Autodesk Inventor part; units mm, degrees
(part 2 of 2)
sketch "Sketch7" plane through (0, 0, 5.08) normal (0, 0, 1) x (1, 0, 0)
  circle A0 centre (7.62, 538.4546) radius 2.5 projected
  circle A1 centre (7.62, 482.5746) radius 2.5 projected
  line L0 (213.36, 469.8746) -> (213.36, 464.7946) projected
  line L1 (213.36, 464.7946) -> (203.2, 464.7946) projected
  line L2 (203.2, 464.7946) -> (203.2, 469.8746) projected
  line L3 (203.2, 469.8746) -> (213.36, 469.8746) projected
  line L4 (172.72, 469.8746) -> (172.72, 464.7946) projected
  line L5 (172.72, 464.7946) -> (162.56, 464.7946) projected
  line L6 (162.56, 464.7946) -> (162.56, 469.8746) projected
  line L7 (162.56, 469.8746) -> (172.72, 469.8746) projected
  line L8 (193.04, 469.8746) -> (193.04, 464.7946) projected
  line L9 (193.04, 464.7946) -> (182.88, 464.7946) projected
  line L10 (182.88, 464.7946) -> (182.88, 469.8746) projected
  line L11 (182.88, 469.8746) -> (193.04, 469.8746) projected
  line L12 (233.68, 469.8746) -> (233.68, 464.7946) projected
  line L13 (233.68, 464.7946) -> (223.52, 464.7946) projected
  line L14 (223.52, 464.7946) -> (223.52, 469.8746) projected
  line L15 (223.52, 469.8746) -> (233.68, 469.8746) projected
  line L16 (228.6, 71.1074) -> (223.52, 71.1074) projected
  line L17 (228.6, 60.9474) -> (228.6, 71.1074) projected
  line L18 (223.52, 60.9474) -> (228.6, 60.9474) projected
  line L19 (223.52, 60.9474) -> (223.52, 50.7874) projected
  line L20 (228.6, 50.7874) -> (223.52, 50.7874) projected
  line L21 (228.6, 40.6274) -> (228.6, 50.7874) projected
  line L22 (223.52, 40.6274) -> (228.6, 40.6274) projected
  line L23 (223.52, 40.6274) -> (223.52, 30.4674) projected
  line L24 (228.6, 30.4674) -> (223.52, 30.4674) projected
  line L25 (228.6, 20.3074) -> (228.6, 30.4674) projected
  line L26 (223.52, 20.3074) -> (228.6, 20.3074) projected
  line L27 (223.52, 20.3074) -> (223.52, 10.1474) projected
  line L28 (228.6, 10.1474) -> (223.52, 10.1474) projected
  line L29 (228.6, 0) -> (228.6, 10.1474) projected
  line L30 (228.6, 0) -> (309.88, 0) projected
  line L31 (309.88, 10.1474) -> (309.88, 0) projected
  line L32 (314.96, 10.1474) -> (309.88, 10.1474) projected
  line L33 (314.96, 10.1474) -> (314.96, 20.3074) projected
  line L34 (309.88, 20.3074) -> (314.96, 20.3074) projected
  line L35 (309.88, 30.4674) -> (309.88, 20.3074) projected
  line L36 (314.96, 30.4674) -> (309.88, 30.4674) projected
  line L37 (314.96, 30.4674) -> (314.96, 40.6274) projected
  line L38 (309.88, 40.6274) -> (314.96, 40.6274) projected
  line L39 (309.88, 50.7874) -> (309.88, 40.6274) projected
  line L40 (314.96, 50.7874) -> (309.88, 50.7874) projected
  line L41 (314.96, 50.7874) -> (314.96, 60.9474) projected
  line L42 (309.88, 60.9474) -> (314.96, 60.9474) projected
  line L43 (309.88, 71.1074) -> (309.88, 60.9474) projected
  line L44 (314.96, 71.1074) -> (309.88, 71.1074) projected
  line L45 (314.96, 71.1074) -> (314.96, 81.2674) projected
  line L46 (314.96, 81.2674) -> (309.88, 81.2674) projected
  line L47 (309.88, 81.2674) -> (309.88, 91.4274) projected
  line L48 (309.88, 91.4274) -> (314.96, 91.4274) projected
  line L49 (314.96, 91.4274) -> (314.96, 101.5874) projected
  line L50 (314.96, 101.5874) -> (309.88, 101.5874) projected
  line L51 (309.88, 101.5874) -> (309.88, 111.7474) projected
  line L52 (309.88, 111.7474) -> (314.96, 111.7474) projected
  line L53 (314.96, 111.7474) -> (314.96, 121.9074) projected
  line L54 (314.96, 121.9074) -> (309.88, 121.9074) projected
  line L55 (309.88, 121.9074) -> (309.88, 132.0674) projected
  line L56 (309.88, 132.0674) -> (314.96, 132.0674) projected
  line L57 (314.96, 132.0674) -> (314.96, 142.2274) projected
  line L58 (314.96, 142.2274) -> (309.88, 142.2274) projected
  line L59 (309.88, 142.2274) -> (309.88, 152.3874) projected
  line L60 (309.88, 152.3874) -> (314.96, 152.3874) projected
  line L61 (314.96, 152.3874) -> (314.96, 162.5474) projected
  line L62 (314.96, 162.5474) -> (309.88, 162.5474) projected
  line L63 (309.88, 162.5474) -> (309.88, 172.7074) projected
  line L64 (309.88, 172.7074) -> (314.96, 172.7074) projected
  line L65 (314.96, 172.7074) -> (314.96, 182.8674) projected
  line L66 (314.96, 182.8674) -> (309.88, 182.8674) projected
  line L67 (309.88, 182.8674) -> (309.88, 193.0274) projected
  line L68 (309.88, 193.0274) -> (314.96, 193.0274) projected
  line L69 (314.96, 193.0274) -> (314.96, 203.1874) projected
  line L70 (314.96, 203.1874) -> (309.88, 203.1874) projected
  line L71 (309.88, 203.1874) -> (309.88, 213.3474) projected
  line L72 (309.88, 213.3474) -> (314.96, 213.3474) projected
  line L73 (314.96, 213.3474) -> (314.96, 223.5074) projected
  line L74 (314.96, 223.5074) -> (309.88, 223.5074) projected
  line L75 (309.88, 223.5074) -> (309.88, 233.6674) projected
  line L76 (309.88, 233.6674) -> (314.96, 233.6674) projected
  line L77 (314.96, 233.6674) -> (314.96, 243.8274) projected
  line L78 (314.96, 243.8274) -> (309.88, 243.8274) projected
  line L79 (309.88, 243.8274) -> (309.88, 253.9874) projected
  line L80 (309.88, 253.9874) -> (314.96, 253.9874) projected
  line L81 (314.96, 253.9874) -> (314.96, 264.1474) projected
  line L82 (314.96, 264.1474) -> (309.88, 264.1474) projected
  line L83 (309.88, 264.1474) -> (309.88, 274.3074) projected
  line L84 (309.88, 274.3074) -> (314.96, 274.3074) projected
  line L85 (314.96, 274.3074) -> (314.96, 284.4674) projected
  line L86 (314.96, 284.4674) -> (309.88, 284.4674) projected
  line L87 (309.88, 284.4674) -> (309.88, 294.6274) projected
  line L88 (309.88, 294.6274) -> (314.96, 294.6274) projected
  line L89 (314.96, 294.6274) -> (314.96, 304.7874) projected
  line L90 (314.96, 304.7874) -> (309.88, 304.7874) projected
  line L91 (309.88, 304.7874) -> (309.88, 314.9474) projected
  line L92 (309.88, 314.9474) -> (314.96, 314.9474) projected
  line L93 (314.96, 314.9474) -> (314.96, 325.1074) projected
  line L94 (314.96, 325.1074) -> (309.88, 325.1074) projected
  line L95 (309.88, 325.1074) -> (309.88, 335.2674) projected
  line L96 (309.88, 335.2674) -> (314.96, 335.2674) projected
  line L97 (314.96, 335.2674) -> (314.96, 345.4274) projected
  line L98 (314.96, 345.4274) -> (309.88, 345.4274) projected
  line L99 (309.88, 345.4274) -> (309.88, 355.5874) projected
  line L100 (309.88, 355.5874) -> (314.96, 355.5874) projected
  line L101 (314.96, 355.5874) -> (314.96, 365.7474) projected
  line L102 (314.96, 365.7474) -> (309.88, 365.7474) projected
  line L103 (309.88, 365.7474) -> (309.88, 375.9074) projected
  line L104 (309.88, 375.9074) -> (314.96, 375.9074) projected
  line L105 (314.96, 375.9074) -> (314.96, 386.0674) projected
  line L106 (314.96, 386.0674) -> (309.88, 386.0674) projected
  line L107 (309.88, 386.0674) -> (309.88, 396.2274) projected
  line L108 (309.88, 396.2274) -> (314.96, 396.2274) projected
  line L109 (314.96, 396.2274) -> (314.96, 434.1031) projected
  line L110 (314.96, 434.1031) -> (304.1837, 444.8794) projected
  line L111 (304.1837, 444.8794) -> (300.5916, 441.2873) projected
  line L112 (300.5916, 441.2873) -> (293.4074, 448.4715) projected
  line L113 (293.4074, 448.4715) -> (296.9995, 452.0636) projected
  line L114 (296.9995, 452.0636) -> (289.8153, 459.2478) projected
  line L115 (289.8153, 459.2478) -> (286.2232, 455.6557) projected
  line L116 (286.2232, 455.6557) -> (279.039, 462.8399) projected
  line L117 (279.039, 462.8399) -> (282.6311, 466.432) projected
  line L118 (282.6311, 466.432) -> (275.4469, 473.6162) projected
  line L119 (275.4469, 473.6162) -> (271.8548, 470.0241) projected
  line L120 (271.8548, 470.0241) -> (264.6706, 477.2083) projected
  line L121 (264.6706, 477.2083) -> (268.2627, 480.8004) projected
  line L122 (268.2627, 480.8004) -> (261.0785, 487.9847) projected
  line L123 (261.0785, 487.9847) -> (257.4864, 484.3926) projected
  line L124 (257.4864, 484.3926) -> (250.3022, 491.5768) projected
  line L125 (250.3022, 491.5768) -> (253.8943, 495.1689) projected
  line L126 (253.8943, 495.1689) -> (246.7101, 502.3531) projected
  line L127 (246.7101, 502.3531) -> (243.118, 498.761) projected
  line L128 (243.118, 498.761) -> (235.9337, 505.9452) projected
  line L129 (235.9337, 505.9452) -> (239.5258, 509.5373) projected
  line L130 (239.5258, 509.5373) -> (232.3416, 516.7215) projected
  line L131 (232.3416, 516.7215) -> (228.7495, 513.1294) projected
  line L132 (228.7495, 513.1294) -> (221.5653, 520.3136) projected
  line L133 (221.5653, 520.3136) -> (225.1574, 523.9057) projected
  line L134 (225.1574, 523.9057) -> (217.9732, 531.0899) projected
  line L135 (217.9732, 531.0899) -> (214.3811, 527.4978) projected
  line L136 (214.3811, 527.4978) -> (207.1969, 534.682) projected
  line L137 (207.1969, 534.682) -> (210.789, 538.2741) projected
  line L138 (210.789, 538.2741) -> (203.6048, 545.4583) projected
  line L139 (203.6048, 545.4583) -> (200.0127, 541.8662) projected
  line L140 (200.0127, 541.8662) -> (192.8285, 549.0504) projected
  line L141 (192.8285, 549.0504) -> (196.4206, 552.6425) projected
  line L142 (196.4206, 552.6425) -> (193.04, 556.0231) projected
  line L143 (193.04, 556.0231) -> (193.04, 551.1546) projected
  line L144 (193.04, 551.1546) -> (182.88, 551.1546) projected
  line L145 (182.88, 551.1546) -> (182.88, 556.2346) projected
  line L146 (182.88, 556.2346) -> (172.72, 556.2346) projected
  line L147 (172.72, 556.2346) -> (172.72, 551.1546) projected
  line L148 (172.72, 551.1546) -> (162.56, 551.1546) projected
  line L149 (162.56, 551.1546) -> (162.56, 556.2346) projected
  line L150 (162.56, 556.2346) -> (152.4, 556.2346) projected
  line L151 (152.4, 556.2346) -> (152.4, 551.1546) projected
  line L152 (152.4, 551.1546) -> (142.24, 551.1546) projected
  line L153 (142.24, 551.1546) -> (142.24, 556.2346) projected
  line L154 (142.24, 556.2346) -> (132.08, 556.2346) projected
  line L155 (132.08, 556.2346) -> (132.08, 551.1546) projected
  line L156 (132.08, 551.1546) -> (121.92, 551.1546) projected
  line L157 (121.92, 551.1546) -> (121.92, 556.2346) projected
  line L158 (121.92, 556.2346) -> (111.76, 556.2346) projected
  line L159 (111.76, 556.2346) -> (111.76, 551.1546) projected
  line L160 (111.76, 551.1546) -> (101.6, 551.1546) projected
  line L161 (101.6, 551.1546) -> (101.6, 556.2346) projected
  line L162 (101.6, 556.2346) -> (91.44, 556.2346) projected
  line L163 (91.44, 556.2346) -> (91.44, 551.1546) projected
  line L164 (91.44, 551.1546) -> (81.28, 551.1546) projected
  line L165 (81.28, 551.1546) -> (81.28, 556.2346) projected
  line L166 (81.28, 556.2346) -> (71.12, 556.2346) projected
  line L167 (71.12, 556.2346) -> (71.12, 551.1546) projected
  line L168 (71.12, 551.1546) -> (60.96, 551.1546) projected
  line L169 (60.96, 551.1546) -> (60.96, 556.2346) projected
  line L170 (60.96, 556.2346) -> (50.8, 556.2346) projected
  line L171 (50.8, 556.2346) -> (50.8, 551.1546) projected
  line L172 (50.8, 551.1546) -> (40.64, 551.1546) projected
  line L173 (40.64, 551.1546) -> (40.64, 556.2346) projected
  line L174 (40.64, 556.2346) -> (30.48, 556.2346) projected
  line L175 (30.48, 556.2346) -> (30.48, 551.1546) projected
  line L176 (30.48, 551.1546) -> (20.32, 551.1546) projected
  line L177 (20.32, 551.1546) -> (20.32, 556.2346) projected
  line L178 (20.32, 556.2346) -> (10.16, 556.2346) projected
  line L179 (10.16, 556.2346) -> (10.16, 551.1546) projected
  line L180 (10.16, 551.1546) -> (-5.08, 551.1546) projected
  line L181 (-5.08, 551.1546) -> (-5.08, 469.8746) projected
  line L182 (-5.08, 469.8746) -> (10.16, 469.8746) projected
  line L183 (10.16, 469.8746) -> (10.16, 464.7946) projected
  line L184 (10.16, 464.7946) -> (20.32, 464.7946) projected
  line L185 (20.32, 464.7946) -> (20.32, 469.8746) projected
  line L186 (20.32, 469.8746) -> (30.48, 469.8746) projected
  line L187 (30.48, 469.8746) -> (30.48, 464.7946) projected
  line L188 (30.48, 464.7946) -> (40.64, 464.7946) projected
  line L189 (40.64, 464.7946) -> (40.64, 469.8746) projected
  line L190 (40.64, 469.8746) -> (50.8, 469.8746) projected
  line L191 (50.8, 469.8746) -> (50.8, 464.7946) projected
  line L192 (50.8, 464.7946) -> (60.96, 464.7946) projected
  line L193 (60.96, 464.7946) -> (60.96, 469.8746) projected
  line L194 (60.96, 469.8746) -> (71.12, 469.8746) projected
  line L195 (71.12, 469.8746) -> (71.12, 464.7946) projected
  line L196 (71.12, 464.7946) -> (81.28, 464.7946) projected
  line L197 (81.28, 464.7946) -> (81.28, 469.8746) projected
  line L198 (81.28, 469.8746) -> (91.44, 469.8746) projected
  line L199 (91.44, 469.8746) -> (91.44, 464.7946) projected
  line L200 (91.44, 464.7946) -> (101.6, 464.7946) projected
  line L201 (101.6, 464.7946) -> (101.6, 469.8746) projected
  line L202 (101.6, 469.8746) -> (111.76, 469.8746) projected
  line L203 (111.76, 469.8746) -> (111.76, 464.7946) projected
  line L204 (111.76, 464.7946) -> (121.92, 464.7946) projected
  line L205 (121.92, 464.7946) -> (121.92, 469.8746) projected
  line L206 (121.92, 469.8746) -> (132.08, 469.8746) projected
  line L207 (132.08, 469.8746) -> (132.08, 464.7946) projected
  line L208 (132.08, 464.7946) -> (142.24, 464.7946) projected
  line L209 (142.24, 464.7946) -> (142.24, 469.8746) projected
  line L210 (142.24, 469.8746) -> (152.4, 469.8746) projected
  line L211 (152.4, 469.8746) -> (152.4, 464.7946) projected
  line L212 (152.4, 464.7946) -> (154.9528, 464.7946) projected
  line L213 (154.9528, 464.7946) -> (223.52, 396.2274) projected
  line L214 (223.52, 396.2274) -> (228.6, 396.2274) projected
  line L215 (228.6, 396.2274) -> (228.6, 386.0674) projected
  line L216 (228.6, 386.0674) -> (223.52, 386.0674) projected
  line L217 (223.52, 386.0674) -> (223.52, 375.9074) projected
  line L218 (223.52, 375.9074) -> (228.6, 375.9074) projected
  line L219 (228.6, 375.9074) -> (228.6, 365.7474) projected
  line L220 (228.6, 365.7474) -> (223.52, 365.7474) projected
  line L221 (223.52, 365.7474) -> (223.52, 355.5874) projected
  line L222 (223.52, 355.5874) -> (228.6, 355.5874) projected
  line L223 (228.6, 355.5874) -> (228.6, 345.4274) projected
  line L224 (228.6, 345.4274) -> (223.52, 345.4274) projected
  line L225 (223.52, 345.4274) -> (223.52, 335.2674) projected
  line L226 (223.52, 335.2674) -> (228.6, 335.2674) projected
  line L227 (228.6, 335.2674) -> (228.6, 325.1074) projected
  line L228 (228.6, 325.1074) -> (223.52, 325.1074) projected
  line L229 (223.52, 325.1074) -> (223.52, 314.9474) projected
  line L230 (223.52, 314.9474) -> (228.6, 314.9474) projected
  line L231 (228.6, 314.9474) -> (228.6, 304.7874) projected
  line L232 (228.6, 304.7874) -> (223.52, 304.7874) projected
  line L233 (223.52, 304.7874) -> (223.52, 294.6274) projected
  line L234 (223.52, 294.6274) -> (228.6, 294.6274) projected
  line L235 (228.6, 294.6274) -> (228.6, 284.4674) projected
  line L236 (228.6, 284.4674) -> (223.52, 284.4674) projected
  line L237 (223.52, 284.4674) -> (223.52, 274.3074) projected
  line L238 (223.52, 274.3074) -> (228.6, 274.3074) projected
  line L239 (228.6, 274.3074) -> (228.6, 264.1474) projected
  line L240 (228.6, 264.1474) -> (223.52, 264.1474) projected
  line L241 (223.52, 264.1474) -> (223.52, 253.9874) projected
  line L242 (223.52, 253.9874) -> (228.6, 253.9874) projected
  line L243 (228.6, 253.9874) -> (228.6, 243.8274) projected
  line L244 (228.6, 243.8274) -> (223.52, 243.8274) projected
  line L245 (223.52, 243.8274) -> (223.52, 233.6674) projected
  line L246 (223.52, 233.6674) -> (228.6, 233.6674) projected
  line L247 (228.6, 233.6674) -> (228.6, 223.5074) projected
  line L248 (228.6, 223.5074) -> (223.52, 223.5074) projected
  line L249 (223.52, 223.5074) -> (223.52, 213.3474) projected
  line L250 (223.52, 213.3474) -> (228.6, 213.3474) projected
  line L251 (228.6, 213.3474) -> (228.6, 203.1874) projected
  line L252 (228.6, 203.1874) -> (223.52, 203.1874) projected
  line L253 (223.52, 203.1874) -> (223.52, 193.0274) projected
  line L254 (223.52, 193.0274) -> (228.6, 193.0274) projected
  line L255 (228.6, 193.0274) -> (228.6, 182.8674) projected
  line L256 (228.6, 182.8674) -> (223.52, 182.8674) projected
  line L257 (223.52, 182.8674) -> (223.52, 172.7074) projected
  line L258 (223.52, 172.7074) -> (228.6, 172.7074) projected
  line L259 (228.6, 172.7074) -> (228.6, 162.5474) projected
  line L260 (228.6, 162.5474) -> (223.52, 162.5474) projected
  line L261 (223.52, 162.5474) -> (223.52, 152.3874) projected
  line L262 (223.52, 152.3874) -> (228.6, 152.3874) projected
  line L263 (228.6, 152.3874) -> (228.6, 142.2274) projected
  line L264 (228.6, 142.2274) -> (223.52, 142.2274) projected
  line L265 (223.52, 142.2274) -> (223.52, 132.0674) projected
  line L266 (223.52, 132.0674) -> (228.6, 132.0674) projected
  line L267 (228.6, 132.0674) -> (228.6, 121.9074) projected
  line L268 (228.6, 121.9074) -> (223.52, 121.9074) projected
  line L269 (223.52, 121.9074) -> (223.52, 111.7474) projected
  line L270 (223.52, 111.7474) -> (228.6, 111.7474) projected
  line L271 (228.6, 111.7474) -> (228.6, 101.5874) projected
  line L272 (228.6, 101.5874) -> (223.52, 101.5874) projected
  line L273 (223.52, 101.5874) -> (223.52, 91.4274) projected
  line L274 (223.52, 91.4274) -> (228.6, 91.4274) projected
  line L275 (228.6, 91.4274) -> (228.6, 81.2674) projected
  line L276 (228.6, 81.2674) -> (223.52, 81.2674) projected
  line L277 (223.52, 81.2674) -> (223.52, 71.1074) projected
  line L278 (-5.08, 469.8746) -> (0, 469.8746)
  line L279 (0, 469.8746) -> (0, 464.7946)
  line L280 (0, 464.7946) -> (-5.08, 464.7946)
  line L281 (-5.08, 464.7946) -> (-5.08, 469.8746)
  line L282 (162.56, 469.8746) -> (233.68, 469.8746)
  line L283 (233.68, 469.8746) -> (233.68, 464.7946)
  line L284 (233.68, 464.7946) -> (162.56, 464.7946)
  line L285 (162.56, 464.7946) -> (162.56, 469.8746)
  line L286 (193.04, 556.2346) -> (162.56, 556.2346)
  line L287 (162.56, 556.2346) -> (162.56, 551.1546)
  line L288 (162.56, 551.1546) -> (193.04, 551.1546)
  line L289 (193.04, 551.1546) -> (193.04, 556.0231)
  line L290 (-5.08, 551.1546) -> (0, 551.1546)
  line L291 (0, 551.1546) -> (0, 556.2346)
  line L292 (0, 556.2346) -> (-5.08, 556.2346)
  line L293 (-5.08, 556.2346) -> (-5.08, 551.1546)
  line L294 (162.56, 556.2346) -> (152.4, 556.2346) projected
  line L295 (193.04, 556.2346) -> (193.04, 551.1546)
  point P0 (0, 0)
  dimension "d77" = 5.08
  dimension "d78" = 5.08
  dimension "d79" = 5.08
  dimension "d80" = 5.08
  constraints: 34 end point, 8 parallel, 4 horizontal, 4 perpendicular, 1 collinear, 1 vertical
  measures "d77" distance of L279.end L280.end
  measures "d78" distance of L278.end L279.end
  measures "d79" distance of L292.end L291.end
  measures "d80" distance of L291.end L290.end
extrude "Extrusion5" add sketch "Sketch7" against normal blind 5.08 contours L0 L1 L2 L3 | L15 L12 L13 L14 | L8 L9 L10 L11 | L4 L5 L6 L7 | L16 L277 L276 L275 L274 L273 L272 L271 L270 L269 L268 L267 L266 L265 L264 L263 L262 L261 L260 L259 L258 L257 L256 L255 L254 L253 L252 L251 L250 L249 L248 L247 L246 L245 L244 L243 L242 L241 L240 L239 L238 L237 L236 L235 L234 L233 L232 L231 L230 L229 L228 L227 L226 L225 L224 L223 L222 L221 L220 L219 L218 L217 L216 L215 L214 L213 L212 L211 L210 L209 L208 L207 L206 L205 L204 L203 L202 L201 L200 L199 L198 L197 L196 L195 L194 L193 L192 L191 L190 L189 L188 L187 L186 L185 L184 L183 L182 L181 L180 L179 L178 L177 L176 L175 L174 L173 L172 L171 L170 L169 L168 L167 L166 L165 L164 L163 L162 L161 L160 L159 L158 L157 L156 L155 L154 L153 L152 L151 L150 L149 L148 L288 L144 L143 L142 L141 L140 L139 L138 L137 L136 L135 L134 L133 L132 L131 L130 L129 L128 L127 L126 L125 L124 L123 L122 L121 L120 L119 L118 L117 L116 L115 L114 L113 L112 L111 L110 L109 L108 L107 L106 L105 L104 L103 L102 L101 L100 L99 L98 L97 L96 L95 L94 L93 L92 L91 L90 L89 L88 L87 L86 L85 L84 L83 L82 L81 L80 L79 L78 L77 L76 L75 L74 L73 L72 L71 L70 L69 L68 L67 L66 L65 L64 L63 L62 L61 L60 L59 L58 L57 L56 L55 L54 L53 L52 L51 L50 L49 L48 L47 L46 L45 L44 L43 L42 L41 L40 L39 L38 L37 L36 L35 L34 L33 L32 L31 L30 L29 L28 L27 L26 L25 L24 L23 L22 L21 L20 L19 L18 L17 | L279 L280 L281 L182 | L293 L292 L291 L180 | L143 L144 L145 L286 L295 | L288 L147 L146 L145 | L148 L149 L286 L147
equation "\"d2\" = d0"
equation "\"d4\" = d2"
equation "\"d18\" = 2 * d14"
equation "\"d38\" = 2 * d35"
equation "\"d52\" = 2 * d48"
equation "\"d68\" = d67"
body "Solid1"
